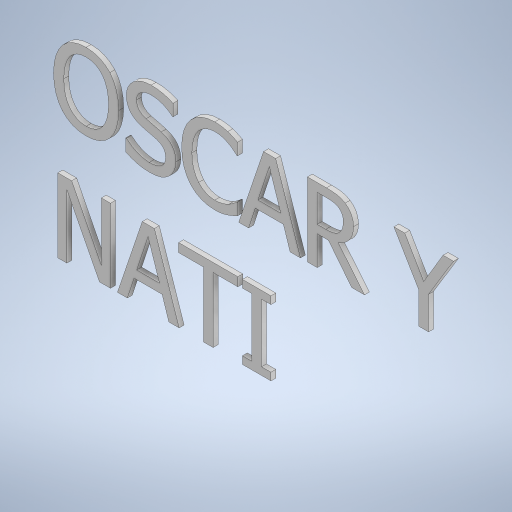
# Autodesk Inventor part: DECORACION
Saved by Autodesk Inventor 2023 (Build 270158000, 158)
## iProperties
Created: 2024-11-28
Part Number: DECORACION
Material: Genérico
Document SubType Name: Modeling
Designer: Osqui Alvareto
Density: 1 g/cm^3
Appearance: Valor por defecto
Author: Osqui Alvareto
Autodesk Inventor part; units mm, degrees
ref_plane "YZ Plane" through (0, 0, 0) normal (1, 0, 0) x (0, 1, 0)
ref_plane "XZ Plane" through (0, 0, 0) normal (0, 1, 0) x (-1, 0, 0)
ref_plane "XY Plane" through (0, 0, 0) normal (0, 0, 1) x (1, 0, 0)
sketch "Boceto1" plane through (0, 0, 0) normal (0, 0, 1) x (1, 0, 0)
  line L0 (0.157, 33.1964) -> (168.99, 33.1964) construction
  line L1 (168.99, 33.1964) -> (168.99, 12.3536) construction
  line L2 (168.99, 12.3536) -> (0.157, 12.3536) construction
  line L3 (0.157, 12.3536) -> (0.157, 33.1964) construction
  spline S0 degree 2 poles (24.4195, 29.1364) (26.1213, 27.1429) (28.0176, 21.3082) (28.0176, 17.5643) knots 0 0 0 1 2 2 2
  spline S1 degree 2 poles (28.0176, 17.5643) (28.0176, 13.9176) (26.1699, 8.01) (24.4195, 6.0165) knots 0 0 0 1 2 2 2
  spline S2 degree 2 poles (24.4195, 6.0165) (22.5719, 3.9257) (17.6853, 1.9322) (14.7437, 1.9322) knots 0 0 0 1 2 2 2
  spline S3 degree 2 poles (14.7437, 1.9322) (11.7048, 1.9322) (6.8426, 3.9987) (5.0678, 6.0165) knots 0 0 0 1 2 2 2
  spline S4 degree 2 poles (5.0678, 6.0165) (3.3417, 8.01) (1.4941, 13.869) (1.4941, 17.5643) knots 0 0 0 1 2 2 2
  spline S5 degree 2 poles (1.4941, 17.5643) (1.4941, 21.3326) (3.3661, 27.07) (5.0921, 29.1364) knots 0 0 0 1 2 2 2
  spline S6 degree 2 poles (5.0921, 29.1364) (6.8426, 31.13) (11.7291, 33.1964) (14.7437, 33.1964) knots 0 0 0 1 2 2 2
  spline S7 degree 2 poles (14.7437, 33.1964) (17.8069, 33.1964) (22.7178, 31.057) (24.4195, 29.1364) knots 0 0 0 1 2 2 2
  spline S8 degree 2 poles (23.8604, 17.5643) (23.8604, 20.5303) (22.5719, 25.1251) (21.405, 26.6324) knots 0 0 0 1 2 2 2
  spline S9 degree 2 poles (21.405, 26.6324) (20.2137, 28.1883) (16.8588, 29.7442) (14.768, 29.7442) knots 0 0 0 1 2 2 2
  spline S10 degree 2 poles (14.768, 29.7442) (12.6043, 29.7442) (9.3466, 28.2369) (8.1067, 26.6324) knots 0 0 0 1 2 2 2
  spline S11 degree 2 poles (8.1067, 26.6324) (6.9155, 25.1008) (5.6513, 20.4817) (5.6513, 17.5643) knots 0 0 0 1 2 2 2
  spline S12 degree 2 poles (5.6513, 17.5643) (5.6513, 11.6567) (10.6108, 5.3844) (14.768, 5.3844) knots 0 0 0 1 2 2 2
  spline S13 degree 2 poles (14.768, 5.3844) (18.9252, 5.3844) (23.8604, 11.6567) (23.8604, 17.5643) knots 0 0 0 1 2 2 2
  spline S14 degree 2 poles (40.7567, 2.0295) (37.499, 2.0295) (32.9285, 3.3909) (30.9106, 4.3633) knots 0 0 0 1 2 2 2
  line L4 (30.9106, 4.3633) -> (30.9106, 9.3715)
  line L5 (30.9106, 9.3715) -> (31.2024, 9.3715)
  spline S15 degree 2 poles (31.2024, 9.3715) (33.1716, 7.5238) (38.1554, 5.4817) (40.4649, 5.4817) knots 0 0 0 1 2 2 2
  spline S16 degree 2 poles (40.4649, 5.4817) (43.7712, 5.4817) (47.1505, 8.2288) (47.1505, 10.4898) knots 0 0 0 1 2 2 2
  spline S17 degree 2 poles (47.1505, 10.4898) (47.1505, 12.2888) (45.3758, 14.5254) (43.4552, 15.0846) knots 0 0 0 1 2 2 2
  spline S18 degree 2 poles (43.4552, 15.0846) (42.0695, 15.4736) (39.7599, 16.0084) (38.0338, 16.446) knots 0 0 0 1 2 2 2
  spline S19 degree 2 poles (38.0338, 16.446) (36.4779, 16.8593) (34.0225, 18.0992) (33.0743, 19.0959) knots 0 0 0 1 2 2 2
  spline S20 degree 2 poles (33.0743, 19.0959) (32.1505, 20.0927) (31.1294, 22.7669) (31.1294, 24.5173) knots 0 0 0 1 2 2 2
  spline S21 degree 2 poles (31.1294, 24.5173) (31.1294, 28.164) (36.8182, 33.0992) (41.2186, 33.0992) knots 0 0 0 1 2 2 2
  spline S22 degree 2 poles (41.2186, 33.0992) (43.7469, 33.0992) (48.2202, 32.1024) (50.1408, 31.1543) knots 0 0 0 1 2 2 2
  line L6 (50.1408, 31.1543) -> (50.1408, 26.3893)
  line L7 (50.1408, 26.3893) -> (49.849, 26.3893)
  spline S23 degree 2 poles (49.849, 26.3893) (48.4147, 27.7021) (43.9414, 29.647) (41.486, 29.647) knots 0 0 0 1 2 2 2
  spline S24 degree 2 poles (41.486, 29.647) (38.7145, 29.647) (35.2866, 27.0457) (35.2866, 24.9306) knots 0 0 0 1 2 2 2
  spline S25 degree 2 poles (35.2866, 24.9306) (35.2866, 23.0343) (37.3045, 20.7734) (39.2007, 20.2629) knots 0 0 0 1 2 2 2
  spline S26 degree 2 poles (39.2007, 20.2629) (40.4649, 19.9225) (44.1359, 19.0473) (45.3515, 18.6826) knots 0 0 0 1 2 2 2
  spline S27 degree 2 poles (45.3515, 18.6826) (48.439, 17.7345) (51.3077, 13.9176) (51.3077, 11.1219) knots 0 0 0 1 2 2 2
  spline S28 degree 2 poles (51.3077, 11.1219) (51.3077, 9.3471) (49.8733, 5.9436) (48.5849, 4.7523) knots 0 0 0 1 2 2 2
  spline S29 degree 2 poles (48.5849, 4.7523) (47.1505, 3.4395) (43.5038, 2.0295) (40.7567, 2.0295) knots 0 0 0 1 2 2 2
  spline S30 degree 2 poles (67.0857, 2.0295) (64.1683, 2.0295) (59.2332, 3.9987) (57.4341, 5.9679) knots 0 0 0 1 2 2 2
  spline S31 degree 2 poles (57.4341, 5.9679) (55.6351, 7.9128) (53.6659, 13.7475) (53.6659, 17.54) knots 0 0 0 1 2 2 2
  spline S32 degree 2 poles (53.6659, 17.54) (53.6659, 21.3082) (55.5865, 26.8998) (57.4098, 28.9663) knots 0 0 0 1 2 2 2
  spline S33 degree 2 poles (57.4098, 28.9663) (59.2088, 30.9841) (64.1197, 33.0992) (67.1586, 33.0992) knots 0 0 0 1 2 2 2
  spline S34 degree 2 poles (67.1586, 33.0992) (68.6659, 33.0992) (71.3158, 32.6616) (72.4341, 32.3212) knots 0 0 0 1 2 2 2
  spline S35 degree 2 poles (72.4341, 32.3212) (73.4066, 32.0052) (75.4244, 31.1056) (76.4212, 30.5708) knots 0 0 0 1 2 2 2
  line L8 (76.4212, 30.5708) -> (76.4212, 25.7572)
  line L9 (76.4212, 25.7572) -> (76.1051, 25.7572)
  spline S36 degree 2 poles (76.1051, 25.7572) (75.5703, 26.2434) (73.9171, 27.6048) (72.7259, 28.2612) knots 0 0 0 1 2 2 2
  spline S37 degree 2 poles (72.7259, 28.2612) (71.5832, 28.8933) (68.8847, 29.6956) (67.1343, 29.6956) knots 0 0 0 1 2 2 2
  spline S38 degree 2 poles (67.1343, 29.6956) (65.2137, 29.6956) (61.7858, 28.1154) (60.4973, 26.6081) knots 0 0 0 1 2 2 2
  spline S39 degree 2 poles (60.4973, 26.6081) (59.2332, 25.0765) (57.8231, 20.433) (57.8231, 17.54) knots 0 0 0 1 2 2 2
  spline S40 degree 2 poles (57.8231, 17.54) (57.8231, 14.4525) (59.3061, 10.0035) (60.5946, 8.4719) knots 0 0 0 1 2 2 2
  spline S41 degree 2 poles (60.5946, 8.4719) (61.8588, 6.989) (65.238, 5.4817) (67.1343, 5.4817) knots 0 0 0 1 2 2 2
  spline S42 degree 2 poles (67.1343, 5.4817) (68.8604, 5.4817) (71.802, 6.3326) (72.9447, 6.9646) knots 0 0 0 1 2 2 2
  spline S43 degree 2 poles (72.9447, 6.9646) (74.0387, 7.5967) (75.6675, 8.9095) (76.1294, 9.3715) knots 0 0 0 1 2 2 2
  line L10 (76.1294, 9.3715) -> (76.4212, 9.3715)
  line L11 (76.4212, 9.3715) -> (76.4212, 4.6065)
  spline S44 degree 2 poles (76.4212, 4.6065) (75.4244, 4.1445) (73.674, 3.2937) (72.4341, 2.9047) knots 0 0 0 1 2 2 2
  spline S45 degree 2 poles (72.4341, 2.9047) (71.1213, 2.4671) (68.8847, 2.0295) (67.0857, 2.0295) knots 0 0 0 1 2 2 2
  line L12 (76.9074, 2.5643) -> (87.0208, 32.5643)
  line L13 (87.0208, 32.5643) -> (91.9317, 32.5643)
  line L14 (91.9317, 32.5643) -> (102.0451, 2.5643)
  line L15 (102.0451, 2.5643) -> (97.8393, 2.5643)
  line L16 (97.8393, 2.5643) -> (95.1165, 10.9517)
  line L17 (95.1165, 10.9517) -> (83.6659, 10.9517)
  line L18 (83.6659, 10.9517) -> (80.943, 2.5643)
  line L19 (80.943, 2.5643) -> (76.9074, 2.5643)
  line L20 (94.0225, 14.3552) -> (89.379, 28.48)
  line L21 (89.379, 28.48) -> (84.7599, 14.3552)
  line L22 (84.7599, 14.3552) -> (94.0225, 14.3552)
  line L23 (128.1067, 2.5643) -> (122.9285, 2.5643)
  line L24 (122.9285, 2.5643) -> (113.4471, 14.5011)
  line L25 (113.4471, 14.5011) -> (108.8766, 14.5011)
  line L26 (108.8766, 14.5011) -> (108.8766, 2.5643)
  line L27 (108.8766, 2.5643) -> (104.8896, 2.5643)
  line L28 (104.8896, 2.5643) -> (104.8896, 32.5643)
  line L29 (104.8896, 32.5643) -> (112.6205, 32.5643)
  spline S46 degree 2 poles (112.6205, 32.5643) (115.1975, 32.5643) (118.674, 32.0052) (120.2542, 30.9841) knots 0 0 0 1 2 2 2
  spline S47 degree 2 poles (120.2542, 30.9841) (121.8344, 29.963) (123.6578, 26.7783) (123.6578, 24.4201) knots 0 0 0 1 2 2 2
  spline S48 degree 2 poles (123.6578, 24.4201) (123.6578, 21.1381) (120.3028, 16.6891) (117.4341, 15.6194) knots 0 0 0 1 2 2 2
  line L30 (117.4341, 15.6194) -> (128.1067, 2.5643)
  spline S49 degree 2 poles (119.5006, 24.104) (119.5006, 25.4168) (118.5768, 27.4347) (117.6043, 28.0911) knots 0 0 0 1 2 2 2
  spline S50 degree 2 poles (117.6043, 28.0911) (116.7534, 28.6502) (114.4925, 29.1121) (112.8393, 29.1121) knots 0 0 0 1 2 2 2
  line L31 (112.8393, 29.1121) -> (108.8766, 29.1121)
  line L32 (108.8766, 29.1121) -> (108.8766, 17.8317)
  line L33 (108.8766, 17.8317) -> (112.3774, 17.8317)
  spline S51 degree 2 poles (112.3774, 17.8317) (114.1035, 17.8317) (116.8507, 18.4395) (117.7988, 19.3877) knots 0 0 0 1 2 2 2
  spline S52 degree 2 poles (117.7988, 19.3877) (118.674, 20.2142) (119.5006, 22.5481) (119.5006, 24.104) knots 0 0 0 1 2 2 2
  line L34 (164.379, 32.5643) -> (154.2413, 15.8382)
  line L35 (154.2413, 15.8382) -> (154.2413, 2.5643)
  line L36 (154.2413, 2.5643) -> (150.2542, 2.5643)
  line L37 (150.2542, 2.5643) -> (150.2542, 15.4249)
  line L38 (150.2542, 15.4249) -> (140.1165, 32.5643)
  line L39 (140.1165, 32.5643) -> (144.5411, 32.5643)
  line L40 (144.5411, 32.5643) -> (152.2721, 19.3633)
  line L41 (152.2721, 19.3633) -> (160.1489, 32.5643)
  line L42 (160.1489, 32.5643) -> (164.379, 32.5643)
  line L43 (24.6627, -46.8299) -> (20.1894, -46.8299)
  line L44 (20.1894, -46.8299) -> (6.9155, -20.9628)
  line L45 (6.9155, -20.9628) -> (6.9155, -46.8299)
  line L46 (6.9155, -46.8299) -> (3.1959, -46.8299)
  line L47 (3.1959, -46.8299) -> (3.1959, -16.8299)
  line L48 (3.1959, -16.8299) -> (8.8604, -16.8299)
  line L49 (8.8604, -16.8299) -> (20.943, -40.5819)
  line L50 (20.943, -40.5819) -> (20.943, -16.8299)
  line L51 (20.943, -16.8299) -> (24.6627, -16.8299)
  line L52 (24.6627, -16.8299) -> (24.6627, -46.8299)
  line L53 (27.5071, -46.8299) -> (37.6205, -16.8299)
  line L54 (37.6205, -16.8299) -> (42.5314, -16.8299)
  line L55 (42.5314, -16.8299) -> (52.6448, -46.8299)
  line L56 (52.6448, -46.8299) -> (48.439, -46.8299)
  line L57 (48.439, -46.8299) -> (45.7161, -38.4425)
  line L58 (45.7161, -38.4425) -> (34.2656, -38.4425)
  line L59 (34.2656, -38.4425) -> (31.5427, -46.8299)
  line L60 (31.5427, -46.8299) -> (27.5071, -46.8299)
  line L61 (44.6221, -35.039) -> (39.9787, -20.9142)
  line L62 (39.9787, -20.9142) -> (35.3596, -35.039)
  line L63 (35.3596, -35.039) -> (44.6221, -35.039)
  line L64 (62.4909, -46.8299) -> (62.4909, -20.3793)
  line L65 (62.4909, -20.3793) -> (52.426, -20.3793)
  line L66 (52.426, -20.3793) -> (52.426, -16.8299)
  line L67 (52.426, -16.8299) -> (76.5427, -16.8299)
  line L68 (76.5427, -16.8299) -> (76.5427, -20.3793)
  line L69 (76.5427, -20.3793) -> (66.4779, -20.3793)
  line L70 (66.4779, -20.3793) -> (66.4779, -46.8299)
  line L71 (66.4779, -46.8299) -> (62.4909, -46.8299)
  line L72 (90.0354, -46.8299) -> (78.4147, -46.8299)
  line L73 (78.4147, -46.8299) -> (78.4147, -43.7667)
  line L74 (78.4147, -43.7667) -> (82.2315, -43.7667)
  line L75 (82.2315, -43.7667) -> (82.2315, -19.8931)
  line L76 (82.2315, -19.8931) -> (78.4147, -19.8931)
  line L77 (78.4147, -19.8931) -> (78.4147, -16.8299)
  line L78 (78.4147, -16.8299) -> (90.0354, -16.8299)
  line L79 (90.0354, -16.8299) -> (90.0354, -19.8931)
  line L80 (90.0354, -19.8931) -> (86.2186, -19.8931)
  line L81 (86.2186, -19.8931) -> (86.2186, -43.7667)
  line L82 (86.2186, -43.7667) -> (90.0354, -43.7667)
  line L83 (90.0354, -43.7667) -> (90.0354, -46.8299)
  point P0 (0, 0)
  constraints: 2 other
extrude "Extrusión1" add sketch "Boceto1" along normal blind 2
